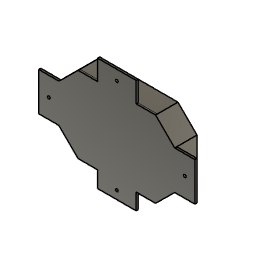
aquarium_base (Autodesk Fusion 360 design; units mm, degrees)
Autodesk Fusion 360 part; units mm, degrees
sketch "Esboço1" plane through (0, 0, 0) normal (0, 1, 0) x (1, 0, 0)
  line L0 (57.25, -4.3166) -> (57.25, -108.6834) construction
  line L1 (114.5, 0) -> (114.5, -113) construction
  line L2 (0, -113) -> (0, 0) construction
  line L3 (57.25, -56.5) -> (-28.25, -56.5) construction
  line L4 (57.25, -56.5) -> (142.75, -56.5) construction
  line L5 (142.75, -56.5) -> (142.75, -85)
  line L6 (142.75, -56.5) -> (142.75, -28)
  line L7 (-28.25, -56.5) -> (-28.25, -85)
  line L8 (-28.25, -56.5) -> (-28.25, -28)
  line L9 (-28.25, -85) -> (0, -113)
  line L10 (114.5, -113) -> (142.75, -85)
  line L11 (114.5, 0) -> (142.75, -28)
  line L12 (0, 0) -> (-28.25, -28)
  line L13 (-28.25, -85) -> (-58.25, -85)
  line L14 (-58.25, -28.2613) -> (-28.25, -28.2613)
  line L15 (-28.25, -28.2613) -> (-28.25, -85)
  line L16 (142.75, -85) -> (172.75, -85)
  line L17 (172.75, -85) -> (172.75, -28)
  line L18 (172.75, -28) -> (142.75, -28)
  line L19 (142.75, -28) -> (142.75, -85)
  line L20 (-48.25, -56.5) -> (-28.25, -56.5) construction
  line L21 (172.75, -56.5) -> (142.75, -56.5) construction
  line L22 (57.25, -4.3166) -> (57.25, 23.9286) construction
  line L23 (57.25, 23.9286) -> (28.75, 23.9286)
  line L24 (28.75, 23.9286) -> (28.75, 0)
  line L25 (57.25, 0) -> (57.25, 23.9286) construction
  line L26 (57.25, 23.9286) -> (85.75, 23.9286)
  line L27 (85.75, 23.9286) -> (85.75, 0)
  line L28 (57.25, 0) -> (57.25, 23.9286) construction
  line L29 (28.75, -113) -> (28.75, -143)
  line L30 (28.75, -143) -> (57.25, -143)
  line L31 (57.25, -137.3166) -> (57.25, -108.6834) construction
  line L32 (114.5, 0) -> (0, 0)
  line L33 (114.5, -113) -> (0, -113)
  line L34 (-58.25, -85) -> (-58.25, -28.2613)
  line L35 (57.25, -143) -> (85.75, -143)
  line L36 (85.75, -143) -> (85.75, -113)
  line L37 (-48.25, -56.5) -> (-58.25, -56.6306) construction
  line L38 (-43.25, -28.2613) -> (-43.25, -85) construction
  circle A0 centre (-43.25, -56.6306) radius 2
  line L39 (85.75, 11.9643) -> (28.75, 11.9643) construction
  circle A1 centre (57.25, 11.9643) radius 2
  line L40 (157.75, -85) -> (157.75, -28) construction
  circle A2 centre (157.75, -56.5) radius 2
  line L41 (85.75, -128) -> (28.75, -128) construction
  circle A3 centre (57.25, -128) radius 2
  dimension "d66" = 113
  dimension "d68" = 85.5
  dimension "d69" = 85.5
  dimension "d74" = 39.7751
  dimension "d75" = 28.5
  dimension "d76" = 28.5
  dimension "d77" = 28.5
  dimension "d78" = 28.5
  dimension "d81" = 30
  dimension "d82" = 30
  dimension "d104" = 28.5
  dimension "d105" = 28.5
  dimension "d107" = 114.5
  dimension "d108" = 28.5
  dimension "d111" = 114.5
  dimension "d112" = 39.7751
  dimension "d113" = 39.7751
  dimension "d114" = 39.7751
  dimension "d115" = 57
  dimension "d121" = 30
  dimension "d122" = 28.5
  dimension "d123" = 30
  dimension "d124" = 30
  dimension "d130" = 4
  dimension "d131" = 4
  dimension "d132" = 4
  dimension "d133" = 4
  constraint coincident L2.end L12.start
  constraint midpoint L0 L3.start
  constraint perpendicular L0 L3
  constraint perpendicular L0 L4
  constraint perpendicular L4 L5
  constraint perpendicular L4 L6
  constraint perpendicular L3 L7
  constraint perpendicular L3 L8
  constraint horizontal L13
  constraint horizontal L14
  constraint vertical L15
  constraint horizontal L16
  constraint vertical L17
  constraint horizontal L18
  constraint vertical L19
  constraint midpoint L17 L21.start
  constraint perpendicular L19 L21
  constraint horizontal L23
  constraint vertical L24
  constraint vertical L25
  constraint horizontal L26
  constraint vertical L27
  constraint vertical L28
  constraint vertical L29
  constraint horizontal L30
  constraint vertical L31
  constraint perpendicular L2 L32
  constraint perpendicular L2 L33
  constraint perpendicular L31 L35
  constraint coincident L33 L36.end
  constraint perpendicular L33 L36
  constraint coincident L33 L29.start
  constraint midpoint L34 L37.end
  constraint midpoint L14 L38.start
  constraint midpoint L13 L38.end
  constraint midpoint L38 A0.centre
  constraint coincident L32 L27.end
  constraint coincident L32 L24.end
  constraint midpoint L27 L39.start
  constraint midpoint L24 L39.end
  constraint midpoint L25 A1.centre
  constraint midpoint L16 L40.start
  constraint midpoint L18 L40.end
  constraint midpoint L21 A2.centre
  constraint midpoint L36 L41.start
  constraint midpoint L29 L41.end
  constraint midpoint L41 A3.centre
  measures "d66" distance of L1.start L1.end
  measures "d68" distance of L3.start L3.end
  measures "d69" distance of L3.start L4.end
  measures "d74" distance of L1.start L6.end
  measures "d75" distance of L3.end L8.end
  measures "d76" distance of L3.end L7.end
  measures "d77" distance of L4.end L5.end
  measures "d78" distance of L4.end L6.end
  measures "d81" distance of L7.end L13.end
  measures "d82" distance of L5.end L16.end
  measures "d104" distance of L22.end L23.end
  measures "d105" distance of L22.end L26.end
  measures "d107" distance of L1.start L2.end
  measures "d108" distance of L29.end L30.end
  measures "d111" distance of L1.end L2.start
  measures "d112" distance of L1.end L5.end
  measures "d113" distance of L2.start L7.end
  measures "d114" distance of L8.end L2.end
  measures "d115" distance of L16.end L17.end
  measures "d121" distance of L14.start L14.end
  measures "d122" distance of L30.end L35.end
  measures "d123" distance of L35.end L36.end
  measures "d124" distance of L29.end L29.start
  measures "d130" diameter of A0
  measures "d131" diameter of A1
  measures "d132" diameter of A2
  measures "d133" diameter of A3
extrude "Extrusão2" add sketch "Esboço1" along normal blind 2 contours L5 L6 L7 L8 L9 L10 L11 L12 L15 L19 L32 L33 makes body 1
extrude "Extrusão3" add sketch "Esboço1" along normal blind 30 thin wall 3 inside separate body contours L5 L6 L7 L8 L9 L10 L11 L12 L15 L19 L32 L33 makes body 2
extrude "Extrusão4" add sketch "Esboço1" against normal blind 3 contours L5 L6 L16 L17 L18 L19 | L5 L6 L7 L8 L9 L10 L11 L12 L15 L19 L32 L33 | L7 L8 L13 L14 L15 L34 | A0 | A2 bodies 2
extrude "Extrusão5" add sketch "Esboço1" along normal blind 30 thin wall 1 inside separate body contours L5 L6 L7 L8 L9 L10 L11 L12 L15 L19 L32 L33 makes body 3
extrude "Extrusão6" add sketch "Esboço1" against normal blind 3 contours L5 L6 L16 L17 L18 L19 | L5 L6 L7 L8 L9 L10 L11 L12 L15 L19 L32 L33 | L29 L30 L33 L35 L36 | L23 L24 L26 L27 L32 | L7 L8 L13 L14 L15 L34 | A0 | A1 | A2 | A3 bodies 3
extrude "Extrusão7" add sketch "Esboço1" along normal blind 30 thin wall 1 inside separate body contours L5 L6 L7 L8 L9 L10 L11 L12 L15 L19 L32 L33 makes body 4
extrude "Extrusão8" add sketch "Esboço1" against normal blind 3 contours L5 L6 L16 L17 L18 L19 | L5 L6 L7 L8 L9 L10 L11 L12 L15 L19 L32 L33 | L29 L30 L33 L35 L36 | L23 L24 L26 L27 L32 | L7 L8 L13 L14 L15 L34 | A0 | A1 | A2 | A3 bodies 4
extrude "Extrusão9" add sketch "Esboço1" along normal blind 30 thin wall 1 inside separate body contours L5 L6 L7 L8 L9 L10 L11 L12 L15 L19 L32 L33 makes body 5
extrude "Extrusão10" add sketch "Esboço1" against normal blind 3 bodies 5
hidden bodies 1 2 3 4
